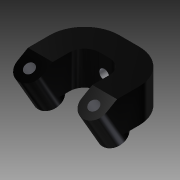
# Autodesk Inventor part: MountB
Saved by Autodesk Inventor 2015 (Build 190159000, 159)
## iProperties
Created: 2017-01-08
Part Number: MountB
Material: Generic
Document SubType Name: Modeling
Designer: Ernest
Density: 1 g/cm^3
Appearance: Default
Mass: 135.561 g
Surface Area: 237.117 cm^2
Volume: 135.561 cm^3
Author: Ernest
Autodesk Inventor part; units mm, degrees
ref_plane "YZ Plane" through (0, 0, 0) normal (1, 0, 0) x (0, 1, 0)
ref_plane "XZ Plane" through (0, 0, 0) normal (0, 1, 0) x (-1, 0, 0)
ref_plane "XY Plane" through (0, 0, 0) normal (0, 0, 1) x (1, 0, 0)
sketch "Sketch1" plane through (0, 0, 0) normal (0, 0, 1) x (1, 0, 0)
  circle A0 centre (0, 0) radius 5
  circle A1 centre (65, 0) radius 5
  circle A2 centre (0, 0) radius 12.5
  circle A3 centre (65, 0) radius 12.5
  line L0 (22.5, 9.5) -> (42.5, 9.5)
  line L1 (42.5, 9.5) -> (42.5, -10.5)
  line L2 (42.5, -10.5) -> (22.5, -10.5)
  line L3 (22.5, -10.5) -> (22.5, 9.5)
  line L4 (0, 0) -> (65, 0) construction
  line L5 (32.5, 0) -> (32.5, 40) construction
  line L6 (27.5, 40) -> (37.5, 40)
  line L7 (12.5, 0) -> (12.5, 25)
  line L8 (52.5, 0) -> (52.5, 25)
  arc A4 (27.5, 40) -> (12.5, 25) centre (27.5, 25) ccw
  arc A5 (52.5, 25) -> (37.5, 40) centre (37.5, 25) ccw
  line L9 (-12.5, 0) -> (-12.5, 30)
  line L10 (77.5, 0) -> (77.5, 30)
  line L11 (22.5, 65) -> (42.5, 65)
  arc A6 (22.5, 65) -> (-12.5, 30) centre (22.5, 30) ccw
  arc A7 (77.5, 30) -> (42.5, 65) centre (42.5, 30) ccw
  point P0 (22.5, 40)
  point P1 (42.5, 40)
  dimension "d0" = 10
  dimension "d1" = 10
  dimension "d2" = 65
  dimension "d3" = 25
  dimension "d4" = 25
  dimension "d5" = 22.5
  dimension "d6" = 22.5
  dimension "d7" = 9.5
  dimension "d8" = 10.5
  dimension "d11" = 20
  dimension "d12" = 10
  dimension "d13" = 40
  dimension "d14" = 15
  dimension "d15" = 65
  dimension "d16" = 35
  constraints: 24 end point, 12 point on circle, 12 tangent, 8 centre point, 4 horizontal, 4 point on line, 3 coincident, 3 perpendicular, 3 vertical, 2 equal radius, 2 midpoint, 2 parallel
  measures "d0" diameter of A0
  measures "d1" diameter of A1
  measures "d2" distance of A1.centre point (0, 0)
  measures "d3" diameter of A2
  measures "d4" diameter of A3
  measures "d5" distance from line of L3 point (0, 0)
  measures "d6" distance from line of L1 A1.centre
  measures "d7" distance from line of L0 point (0, 0)
  measures "d8" distance from line of point (0, 0) L2
  measures "d11" distance of point (22.5, 40) point (42.5, 40)
  measures "d12" distance of L5.end point (22.5, 40)
  measures "d13" distance of L5.start L5.end
  measures "d14" radius of A4
  measures "d15" distance from line of L11 L5.start
  measures "d16" radius of A6
extrude "Extrusion1" add sketch "Sketch1" along normal blind 34 contours A0 | A1 | A2 | A2 L9 A6 L11 A7 L10 A3 L8 A5 L6 A4 L7 | A3
ref_plane "Work Plane4" through (42.5, 65, 0) normal (0, 0.5, -0.8660254) x (-1, 0, 0)
sketch "Sketch17" plane through (42.5, 65, 0) normal (0, 0.5, -0.8660254) x (-1, 0, 0)
  ellipse E0 centre (42.5, -39.2917) end of major axis (30, -39.2917) minor radius 10.8253 (30, -39.2917) -> (55, -39.2917) ccw projected
  line L0 (30, -39.2917) -> (30, -17.641) projected
  ellipse E1 centre (15, -17.641) end of major axis (30, -17.641) minor radius 12.9904 (30, -17.641) -> (15, -4.6506) ccw projected
  line L1 (15, -4.6506) -> (5, -4.6506) projected
  ellipse E2 centre (5, -17.641) end of major axis (20, -17.641) minor radius 12.9904 (5, -4.6506) -> (-10, -17.641) ccw projected
  line L2 (-10, -17.641) -> (-10, -39.2917) projected
  ellipse E3 centre (-22.5, -39.2917) end of major axis (-35, -39.2917) minor radius 10.8253 (-35, -39.2917) -> (-10, -39.2917) ccw projected
  line L3 (-35, -39.2917) -> (-35, -13.3109) projected
  ellipse E4 centre (0, -13.3109) end of major axis (-35, -13.3109) minor radius 30.3109 (0, 17) -> (-35, -13.3109) ccw projected
  line L4 (0, 17) -> (20, 17) projected
  ellipse E5 centre (20, -13.3109) end of major axis (55, -13.3109) minor radius 30.3109 (55, -13.3109) -> (20, 17) ccw projected
  line L5 (55, -13.3109) -> (55, -39.2917) projected
  circle A0 centre (-22.5, -45.117) radius 5
  circle A1 centre (42.5, -45.117) radius 5
  circle A2 centre (-22.5, -45.117) radius 12.5
  circle A3 centre (42.5, -45.117) radius 12.5
  point P0 (42.5, -56.2917)
  dimension "d83" = 10
  dimension "d84" = 10
  dimension "d85" = 25
  dimension "d86" = 25
  constraints: 4 centre point, 2 coincident, 8 other
  measures "d83" diameter of A0
  measures "d84" diameter of A1
  measures "d85" diameter of A2
  measures "d86" diameter of A3
extrude "Extrusion21" cut sketch "Sketch17" against normal blind 75.25 contours A1 | A0
extrude "Extrusion22" add sketch "Sketch17" against normal blind 58 contours A3 E0 | E0 A3 | A2 E3 | E3 A2
extrude "Extrusion23" cut sketch "Sketch17" against normal blind 18.75 contours A3 E0 | E0 A3 | A2 E3 | E3 A2
sketch "Sketch18" plane through (77.5, 0, 34) normal (1, 0, 0) x (0, 0, -1)
  line L0 (5.5058, -1.6465) -> (5.5058, -1.6465) projected
  line L1 (5.5058, -1.6465) -> (5.5058, -1.6465) projected
  line L2 (13.0716, -14.751) -> (-1.0767, 9.7546)
  line L3 (5.5058, -1.6465) -> (12.579, -13.8978) projected
  line L4 (-1.0767, 9.7546) -> (-15.741, 1.2882)
  line L5 (-15.741, 1.2882) -> (-1.5927, -23.2175)
  line L6 (-1.5927, -23.2175) -> (13.0716, -14.751)
  point P0 (34, 0)
  constraints: 8 end point, 3 perpendicular, 1 collinear
extrude "Extrusion24" cut sketch "Sketch18" against normal blind 107.25
sketch "Sketch19" plane through (65, 16.5526, -6.3205) normal (0, 0.5, -0.8660254) x (-1, 0, 0)
  circle A0 centre (0, 0) radius 5 projected
  circle A1 centre (0, 0) radius 12.5 projected
  circle A2 centre (65, 0) radius 5 projected
  circle A3 centre (65, 0) radius 12.5 projected
  line L0 (-12.5, 0) -> (-17.2667, 0)
  line L1 (-17.2667, 0) -> (-17.2667, -28.7026)
  line L2 (-17.2667, -28.7026) -> (21.0012, -28.7026)
  line L3 (21.0012, -28.7026) -> (21.0012, 0)
  line L4 (21.0012, 0) -> (12.5, 0)
  line L5 (52.5, 0) -> (49.0235, 0)
  line L6 (49.0235, 0) -> (49.0235, -27.0388)
  line L7 (49.0235, -27.0388) -> (85.6276, -27.0388)
  line L8 (85.6276, -27.0388) -> (85.6276, 0)
  line L9 (85.6276, 0) -> (77.5, 0)
  circle A4 centre (0, 0) radius 12.5
  circle A5 centre (65, 0) radius 12.5
  point P0 (65, -11.1747)
  constraints: 20 end point, 6 perpendicular, 5 point on line, 2 centre point, 2 coincident, 2 point on circle, 1 concentric, 1 horizontal
extrude "Extrusion25" cut sketch "Sketch19" against normal blind 107.25 contours L4 L3 L2 L1 L0 A1 | L9 L8 L7 L6 L5 A3
sketch "Sketch20" plane through (22.5, 65, 0) normal (0, 1, 0) x (1, 0, 0)
  line L0 (20, 0) -> (0, 0) projected
  line L1 (0, 0) -> (0, -34) projected
  line L2 (20, -34) -> (0, -34) projected
  line L3 (20, 0) -> (20, -34) projected
  circle A0 centre (10, -17) radius 5
  point P0 (-22.5, 0)
  dimension "d97" = 10
  dimension "d98" = 20
  dimension "d99" = 34
  dimension "d100" = 17
  dimension "d101" = 10
  constraints: 1 centre point
  measures "d97" diameter of A0
  measures "d98" distance of L0.start L0.end
  measures "d99" distance of L0.end L1.end
  measures "d100" distance from line of L0 A0.centre
  measures "d101" distance from line of L1 A0.centre
extrude "Extrusion26" cut sketch "Sketch20" against normal blind 107.25 contours A0
sketch "Sketch21" plane through (77.5, 30, 34) normal (1, 0, 0) x (0, 0, -1)
  line L0 (11.6506, -30) -> (34, -17.0966) projected
  line L1 (34, -17.0966) -> (34, 0) projected
  line L2 (34, 0) -> (0, 0) projected
  line L3 (0, -22.1103) -> (0, 0) projected
  line L4 (0, -22.1103) -> (4.5551, -30) projected
  line L5 (11.6506, -30) -> (4.5551, -30) projected
  line L6 (11.6506, -30) -> (34, -17.0966) projected
  line L7 (16.305, -27.3128) -> (6.329, -33.0724)
  line L8 (3.829, -28.7423) -> (8.829, -37.4026) projected
  line L9 (0, -22.1103) -> (4.5551, -30) projected
  line L10 (3.7024, -28.5229) -> (13.6783, -22.7633)
  line L11 (13.6783, -22.7633) -> (16.305, -27.3128)
  point P0 (34, -30)
  constraints: 6 end point, 2 point on line, 1 midpoint, 1 parallel, 1 perpendicular
extrude "Extrusion27" add sketch "Sketch21" against normal blind 90 contours L5 L4 L10 L11 L0 | L7 L8 L5
sketch "Sketch22" plane through (65, 16.5526, -6.3205) normal (0, 0.5, -0.8660254) x (-1, 0, 0)
  circle A0 centre (0, 0) radius 5 projected
  circle A1 centre (0, 0) radius 12.5 projected
  circle A2 centre (65, 0) radius 5 projected
  circle A3 centre (65, 0) radius 12.5 projected
  arc A4 (77.5, 0) -> (52.5, 0) centre (65, 0) ccw projected
  line L0 (77.5, 14.8061) -> (77.5, 0) projected
  ellipse E0 centre (42.5, 14.8061) end of major axis (77.5, 14.8061) minor radius 30.3109 (77.5, 14.8061) -> (42.5, 45.117) ccw projected
  line L1 (22.5, 45.117) -> (42.5, 45.117) projected
  ellipse E1 centre (22.5, 14.8061) end of major axis (-12.5, 14.8061) minor radius 30.3109 (22.5, 45.117) -> (-12.5, 14.8061) ccw projected
  line L2 (-12.5, 0) -> (-12.5, 14.8061) projected
  arc A5 (12.5, 0) -> (-12.5, 0) centre (0, 0) ccw projected
  line L3 (12.5, 10.476) -> (12.5, 0) projected
  ellipse E2 centre (27.5, 10.476) end of major axis (42.5, 10.476) minor radius 12.9904 (27.5, 23.4663) -> (12.5, 10.476) ccw projected
  line L4 (37.5, 23.4663) -> (27.5, 23.4663) projected
  ellipse E3 centre (37.5, 10.476) end of major axis (52.5, 10.476) minor radius 12.9904 (52.5, 10.476) -> (37.5, 23.4663) ccw projected
  line L5 (52.5, 0) -> (52.5, 10.476) projected
  circle A6 centre (0, 0) radius 5
  circle A7 centre (65, 0) radius 5
  line L6 (12.5, 5.2533) -> (52.5, 5.2533)
  line L7 (52.5, 5.2533) -> (52.5, 0)
  line L8 (52.5, 0) -> (12.5, 0)
  line L9 (12.5, 0) -> (12.5, 5.2533)
  point P0 (65, -11.1747)
  constraints: 8 end point, 2 centre point, 2 coincident, 2 concentric, 2 parallel, 1 horizontal, 1 perpendicular, 4 other
extrude "Extrusion28" cut sketch "Sketch22" against normal blind 90 contours A0 | L3 L6 L5 L8 | L3 E2 L4 E3 L5 L6 | A2
equation "\"d12\" = 0.5 * d11"
equation "\"d15\" = d13 + d3"
equation "\"d100\" = 0.5 * d99"
equation "\"d101\" = 0.5 * d98"
body "Solid1"
